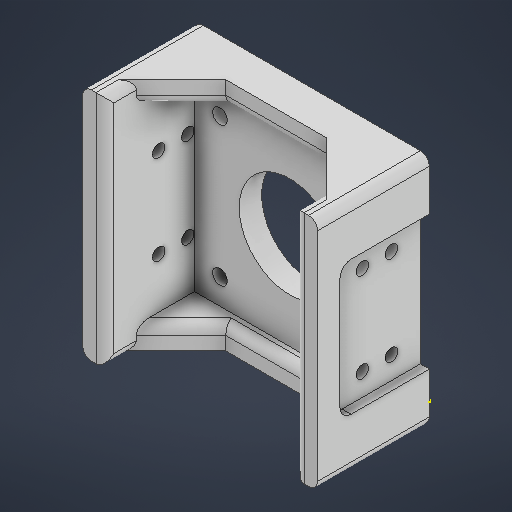
# Autodesk Inventor part: Tool4
Saved by Autodesk Inventor 2027.1 (Build 311270010, 270A)
## iProperties
Created: 2026-08-16
Part Number: Tool4
Material: Generic
Document SubType Name: Sheet Metal
Designer: MSI
Density: 1 g/cm^3
Sheet Metal Rule: Default_mm
Appearance: Default
Author: MSI
Autodesk Inventor part; units mm, degrees
ref_plane "YZ Plane" through (0, 0, 0) normal (1, 0, 0) x (0, 1, 0)
ref_plane "XZ Plane" through (0, 0, 0) normal (0, 1, 0) x (-1, 0, 0)
ref_plane "XY Plane" through (0, 0, 0) normal (0, 0, 1) x (1, 0, 0)
sketch "Sketch1" plane through (0, 0, 0) normal (0, 0, 1) x (1, 0, 0)
  line L0 (0, 0) -> (42.5, 0)
  line L1 (42.5, 0) -> (42.5, 42.5)
  line L2 (42.5, 42.5) -> (0, 42.5)
  line L3 (0, 42.5) -> (0, 0)
  line L4 (-3, 47.5) -> (45.5, 47.5)
  line L5 (47.5, 45.5) -> (47.5, -3)
  line L6 (45.5, -5) -> (-3, -5)
  line L7 (-5, -3) -> (-5, 45.5)
  arc A0 (-3, 47.5) -> (-5, 45.5) centre (-3, 45.5) ccw
  arc A1 (47.5, 45.5) -> (45.5, 47.5) centre (45.5, 45.5) ccw
  arc A2 (45.5, -5) -> (47.5, -3) centre (45.5, -3) ccw
  arc A3 (-5, -3) -> (-3, -5) centre (-3, -3) ccw
  line L8 (0, 21.25) -> (42.5, 21.25)
  line L9 (21.25, 42.5) -> (21.25, 0)
  circle A4 centre (36.8, 36.8) radius 1.65
  circle A5 centre (21.25, 21.25) radius 11.25
  circle A6 centre (5.7, 36.8) radius 1.65
  circle A7 centre (5.7, 5.7) radius 1.65
  circle A8 centre (36.8, 5.7) radius 1.65
  line L10 (0, 42.5) -> (0, 47.5)
  line L11 (0, 0) -> (0, -5)
  line L12 (42.5, 0) -> (42.5, -5)
  line L13 (42.5, 42.5) -> (42.5, 47.5)
  dimension "d0" = 42.5
  dimension "d1" = 42.5
  dimension "d2" = 5
  dimension "d3" = 2
  dimension "d4" = 3.3
  dimension "d5" = 15.55
  dimension "d7" = 15.55
  dimension "d10" = 360
  dimension "d12" = 22.5
  constraints: 28 end point, 9 centre point, 8 point on circle, 8 tangent, 6 point on line, 5 midpoint, 4 parallel, 4 perpendicular, 3 equal radius, 1 horizontal, 12 other
  measures "d0" distance of L2.end L1.end
  measures "d1" distance of L1.end L0.end
  measures "d2" distance between parallel lines of L2 L4
  measures "d3" radius of A0
  measures "d4" diameter of A4
  measures "d5" distance from line of L8 A4.centre
  measures "d7" distance from line of A4.centre L9
  measures "d12" diameter of A5
extrude "Extrusion1" add sketch "Sketch1" along normal blind 25 contours L11 L6 A3 L7 A0 L4 L10 L3 | L1 L13 L4 A1 L5 A2 L6 L12
extrude "Extrusion2" add sketch "Sketch1" along normal blind 5 contours L3 L8 A5 L9 L0 | L9 A5 L8 L1 L0 | L3 L2 L9 A5 L8 | L8 A5 L9 L2 L1
extrude "Extrusion3" add sketch "Sketch1" along normal blind 8 contours L0 L12 L6 L11 | L10 L4 L13 L2
chamfer "Chamfer1" distance 10 angle 45 4 edges at (0, 45, 8) (0, -2.5, 8) (42.5, -2.5, 8) (42.5, 45, 8)
fillet "Fillet1" radius 2 12 edges at (42.5, 21.25, 25) (0, 21.25, 25) (0, 47.5, 21.5) (0, -5, 21.5) (42.5, 47.5, 21.5) (42.5, -5, 21.5) (37.5, 0, 13) (37.5, 42.5, 13) (21.25, 42.5, 8) (21.25, 0, 8) (5, 42.5, 13) (5, 0, 13)
sketch "Sketch2" plane through (47.5, -3, 0) normal (1, 0, 0) x (0, 0, -1)
  point P0 (0, 3)
sketch "Sketch3" plane through (-5, -3, 0) normal (-1, 0, 0) x (0, 0, 1)
  circle A0 centre (13, 34.25) radius 1.4
  circle A1 centre (13, 14.25) radius 1.4
  line L0 (0, 50.5) -> (25, 50.5) projected
  line L1 (0, -2) -> (25, -2) projected
  circle A2 centre (6.5, 34.25) radius 1.4
  circle A3 centre (6.5, 14.25) radius 1.4
  point P0 (0, 3)
  point P1 (12.5, 50.5)
  point P2 (12.5, -2)
  dimension "d23" = 2.8
  dimension "d24" = 2.8
  dimension "d25" = 16.25
  dimension "d26" = 20
  dimension "d27" = 16.25
  dimension "d28" = 2.8
  dimension "d29" = 2.8
  dimension "d30" = 20
  dimension "d31" = 6.5
  constraints: 4 centre point, 2 midpoint
  measures "d23" diameter of A0
  measures "d24" diameter of A1
  measures "d25" vertical distance of point (12.5, 50.5) A0.centre
  measures "d26" distance of A1.centre A0.centre
  measures "d27" vertical distance of point (12.5, -2) A1.centre
  measures "d28" diameter of A2
  measures "d29" diameter of A3
  measures "d30" distance of A3.centre A2.centre
  measures "d31" distance of A1.centre A3.centre
extrude "Extrusion4" cut sketch "Sketch3" against normal blind 5
pattern_circular "Circular Pattern1" count 2 over 360 about axis through (21.25, 21.25, 0) along (0, 0, 1) of "Extrusion4"
sketch "Sketch4" plane through (-5, -3, 0) normal (-1, 0, 0) x (0, 0, 1)
  line L0 (0, 48.5) -> (0, 0) projected
  line L1 (0, 39.25) -> (17.5, 39.25)
  line L2 (20, 36.75) -> (20, 11.75)
  line L3 (17.5, 9.25) -> (0, 9.25)
  circle A0 centre (13, 34.25) radius 1.4 projected
  circle A1 centre (13, 14.25) radius 1.4 projected
  line L4 (0, 39.25) -> (0, 9.25)
  arc A2 (20, 36.75) -> (17.5, 39.25) centre (17.5, 36.75) ccw
  arc A3 (17.5, 9.25) -> (20, 11.75) centre (17.5, 11.75) ccw
  point P0 (0, 3)
  point P1 (20, 9.25)
  dimension "d37" = 5
  dimension "d38" = 5
  dimension "d39" = 20
  dimension "d40" = 2.5
  constraints: 8 end point, 4 point on circle, 4 point on line, 4 tangent, 2 centre point, 2 perpendicular, 1 equal radius, 1 horizontal, 1 vertical
  measures "d37" distance from line of L1 A0.centre
  measures "d38" distance from line of A1.centre L3
  measures "d39" distance of point (20, 9.25) L3.end
  measures "d40" radius of A2
extrude "Extrusion5" cut sketch "Sketch4" against normal blind 2
pattern_circular "Circular Pattern2" count 2 over 360 about axis through (21.25, 21.25, 0) along (0, 0, 1) of "Extrusion5"
body "Solid1"
